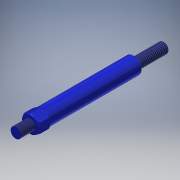
# Autodesk Inventor part: Component 9 (Suspension Spacer)
Saved by Autodesk Inventor 2018 (Build 220112000, 112)
## iProperties
Created: 2023-03-14
Part Number: Component 9 (Suspension Spacer)
Material: Generic
Document SubType Name: Modeling
Designer: Habib Mohamed
Density: 1 g/cm^3
Appearance: Blue - Wall Paint - Glossy
Author: Habib Mohamed
Autodesk Inventor part; units mm, degrees
ref_plane "YZ Plane" through (0, 0, 0) normal (1, 0, 0) x (0, 1, 0)
ref_plane "XZ Plane" through (0, 0, 0) normal (0, 1, 0) x (-1, 0, 0)
ref_plane "XY Plane" through (0, 0, 0) normal (0, 0, 1) x (1, 0, 0)
sketch "Sketch1" plane through (0, 0, 0) normal (0, 0, 1) x (1, 0, 0)
  circle A0 centre (0, 0) radius 4
  line L0 (-4, 2.3094) -> (0, 4.6188)
  line L1 (0, 4.6188) -> (4, 2.3094)
  line L2 (4, 2.3094) -> (4, -2.3094)
  line L3 (4, -2.3094) -> (0, -4.6188)
  line L4 (0, -4.6188) -> (-4, -2.3094)
  line L5 (-4, -2.3094) -> (-4, 2.3094)
  point P0 (-4, 0)
  dimension "d0" = 8
  constraints: 12 end point, 2 coincident, 1 horizontal alignment, 1 midpoint, 15 other
extrude "Extrusion1" add sketch "Sketch1" along normal blind 6
sketch "Sketch2" plane through (0, 0, 6) normal (0, 0, 1) x (1, 0, 0)
  circle A0 centre (0, 0) radius 4 projected
extrude "Extrusion2" cut sketch "Sketch2" against normal blind 6 draft 35 keep common part
extrude "Extrusion3" cut sketch "Sketch1" along normal blind 6 draft 35 contours A0 keep common part
sketch "Sketch3" plane through (0, 0, 0) normal (1, 0, 0) x (0, 1, 0)
  line L0 (0, 0) -> (-3.4641, 0) projected
  line L1 (0, 0) -> (0, -59)
  line L2 (0, -59) -> (2, -59)
  line L3 (2.5, -58.5) -> (2.5, -44)
  line L4 (2.5, -44) -> (4, -44)
  line L5 (4, -44) -> (4, 0)
  line L6 (0, 0) -> (27.6878, 0) construction
  line L7 (3.4641, 0) -> (0, 0) projected
  line L8 (4, 0) -> (0, 0)
  line L9 (2.5, -58.5) -> (2, -59)
  point P0 (2.5, -59)
  dimension "d7" = 4
  dimension "d8" = 2.5
  dimension "d9" = 44
  dimension "d10" = 15
  dimension "d11" = 0.5
  dimension "d12" = 0.5
  constraints: 16 end point, 4 perpendicular, 3 point on line, 1 collinear, 1 horizontal, 1 vertical
  measures "d7" distance between parallel lines of L1 L5
  measures "d8" distance between parallel lines of L1 L3
  measures "d9" distance of L4.end L5.end
  measures "d10" distance of point (2.5, -59) L3.end
  measures "d11" distance of L3.start point (2.5, -59)
  measures "d12" distance of L2.end point (2.5, -59)
revolve "Revolution1" add sketch "Sketch3" angle 360 about axis through (0, 0, 0) along (0, 0, -1)
sketch "Sketch4" plane through (0, 0, 6) normal (0, 0, 1) x (1, 0, 0)
  circle A0 centre (0, 0) radius 2 projected
  circle A1 centre (0, 0) radius 2.5
  point P0 (0, 0)
  dimension "d14" = 5
  constraints: 1 centre point, 1 coincident
  measures "d14" diameter of A1
extrude "Extrusion4" add sketch "Sketch4" along normal blind 7 contours A0 | A1
thread "Thread1" size "M5x0.8" class "6g" standard "ANSI Metric M Profile" full length
thread "Thread2" size "M5x0.8" class "6g" standard "ANSI Metric M Profile" full length
equation "\"d12\" = d11"
body "Solid1"
